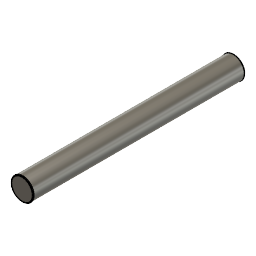
Support Block Shaft (Autodesk Fusion 360 design; units mm, degrees)
part number: 2026-05-14-22-13-12-646
Autodesk Fusion 360 part; units mm, degrees
sketch "Sketch1" plane through (0, 0, 0) normal (0, 0, 1) x (1, 0, 0)
  circle A0 centre (17.78, 17.78) radius 10.795
  dimension "d1" = 21.59
  measures "d1" diameter of A0
extrude "Extrude1" add sketch "Sketch1" along normal blind 25.4 and the other way blind 177.8
chamfer "Chamfer1" distance 0.635 angle 45 2 edges at (7.7155, 13.8764, 25.4) (7.7155, 21.6836, -177.8)
